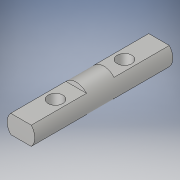
# Autodesk Inventor part: 上昇機構_固定軸ベアリングの
Saved by Autodesk Inventor 2019.4 (Build 234330000, 330)
## iProperties
Created: 2021-12-04
Part Number: 上昇機構_固定軸ベアリングの
Material: アルミニウム 6061
Document SubType Name: Modeling
Designer: 堀川皓史
Density: 2.7 g/cm^3
Appearance: アルミニウム - フラット
Author: 堀川皓史
Autodesk Inventor part; units mm, degrees
ref_plane "YZ Plane" through (0, 0, 0) normal (1, 0, 0) x (0, 1, 0)
ref_plane "XZ Plane" through (0, 0, 0) normal (0, 1, 0) x (-1, 0, 0)
ref_plane "XY Plane" through (0, 0, 0) normal (0, 0, 1) x (1, 0, 0)
sketch "スケッチ1" plane through (0, 0, 0) normal (0, 0, 1) x (1, 0, 0)
  circle A0 centre (0, 0) radius 3
  dimension "d0" = 6
  constraints: 1 centre point, 1 coincident
  measures "d0" diameter of A0
extrude "押し出し1" add sketch "スケッチ1" along normal blind 30
sketch "スケッチ2" plane through (0, 0, 30) normal (0, 0, 1) x (1, 0, 0)
  line L0 (-2.2832, 2) -> (2.2938, 2)
  line L1 (-2.2832, -2) -> (2.3454, -2)
  arc A0 (-2.2361, 2) -> (-2.2361, -2) centre (0, 0) ccw construction
  arc A1 (2.2361, 2) -> (-2.2361, 2) centre (0, 0) ccw
  arc A2 (2.2361, -2) -> (2.2361, 2) centre (0, 0) ccw construction
  arc A3 (-2.2361, -2) -> (2.2361, -2) centre (0, 0) ccw
  dimension "d5" = 2
  dimension "d6" = 6
  dimension "d7" = 2
  constraints: 8 point on circle, 4 centre point, 4 end point, 4 point on line, 2 horizontal, 1 coincident
  measures "d5" distance from line of point (0, 0) L0
  measures "d6" diameter of A0
  measures "d7" distance from line of point (0, 0) L1
extrude "押し出し2" cut sketch "スケッチ2" against normal blind 12
sketch "スケッチ3" plane through (0, 0, 0) normal (0, 0, -1) x (-1, 0, 0)
  arc A0 (-2.2361, -2) -> (2.2361, -2) centre (0, 0) ccw
  line L0 (-2.2361, 2) -> (2.2361, 2)
  line L1 (-2.2361, -2) -> (2.2361, -2)
  arc A1 (2.2361, -2) -> (2.2361, 2) centre (0, 0) ccw construction
  arc A2 (-2.2361, 2) -> (-2.2361, -2) centre (0, 0) ccw construction
  arc A3 (2.2361, 2) -> (-2.2361, 2) centre (0, 0) ccw
  arc A4 (2.2361, -2) -> (2.2361, 2) centre (0, 0) ccw construction
  dimension "d13" = 2
  dimension "d14" = 2
  constraints: 9 point on circle, 4 centre point, 4 end point, 1 coincident, 1 horizontal, 1 parallel
  measures "d13" distance from line of point (0, 0) L0
  measures "d14" distance from line of point (0, 0) L1
extrude "押し出し3" cut sketch "スケッチ3" against normal blind 12
sketch "スケッチ4" plane through (-2.2361, 2, 0) normal (0, 1, 0) x (1, 0, 0)
  circle A0 centre (2.2361, -7.5) radius 1.6
  circle A1 centre (2.2361, -22.5) radius 1.6
  line L0 (0, 0) -> (4.4721, 0) projected
  point P0 (2.2361, 0)
  point P1 (2.2361, 0)
  point P2 (2.2361, 0)
  dimension "d17" = 3.2
  dimension "d18" = 3.2
  dimension "d19" = 15
  dimension "d20" = 7.5
  constraints: 2 centre point, 2 midpoint, 2 vertical alignment
  measures "d17" diameter of A0
  measures "d18" diameter of A1
  measures "d19" distance of A1.centre A0.centre
  measures "d20" distance of point (2.236, 0) A0.centre
extrude "押し出し4" cut sketch "スケッチ4" against normal through all
